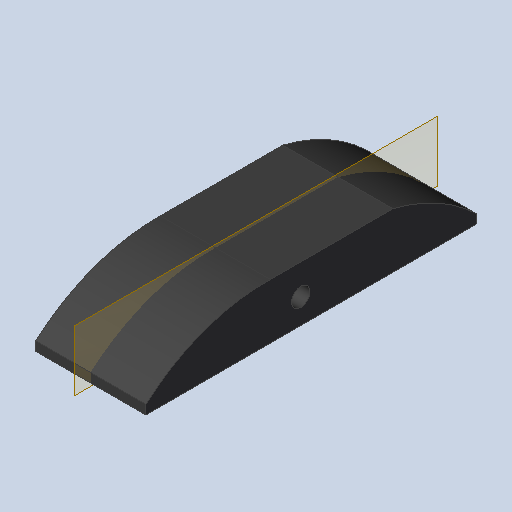
# Autodesk Inventor part: WingBox
Saved by Autodesk Inventor 2025.2 (Build 292293000, 293)
## iProperties
Created: 2025-02-16
Part Number: WingBox
Material: Generic
Document SubType Name: Modeling
Designer: Cupri
Density: 1 g/cm^3
Appearance: Default
Author: Cupri
Autodesk Inventor part; units mm, degrees
ref_plane "YZ Plane" through (0, 0, 0) normal (1, 0, 0) x (0, 1, 0)
ref_plane "XZ Plane" through (0, 0, 0) normal (0, 1, 0) x (-1, 0, 0)
ref_plane "XY Plane" through (0, 0, 0) normal (0, 0, 1) x (1, 0, 0)
sketch "Sketch1" plane through (0, 0, 0) normal (1, 0, 0) x (0, 1, 0)
  line L0 (-38.1, -165.1) -> (-38.1, 165.1)
  line L1 (-38.1, 165.1) -> (20.949, 165.1)
  line L2 (38.1, 77.5498) -> (38.1, -100.5752)
  line L3 (12.4566, -165.1) -> (-38.1, -165.1)
  line L4 (-38.1, -165.1) -> (38.1, 165.1) construction
  line L5 (-38.1, 165.1) -> (38.1, -165.1) construction
  line L6 (-38.1, -165.1) -> (-38.1, -215.9)
  line L7 (-38.1, -215.9) -> (-25.4, -215.9)
  line L8 (-25.4, -215.9) -> (-25.4, -165.1)
  line L9 (-38.1, 165.1) -> (-38.1, 241.3)
  line L10 (-38.1, 241.3) -> (-25.4, 241.3)
  line L11 (-25.4, 241.3) -> (-25.4, 165.1)
  line L12 (-38.1, -139.7) -> (38.1, -139.7) construction
  line L13 (-38.1, 12.7) -> (38.1, 12.7) construction
  line L14 (-38.1, 165.1) -> (38.1, 165.1) construction
  arc A0 (38.1, 68.9574) -> (-25.4, 241.3) centre (-215.8637, 73.2536) ccw
  arc A1 (-25.4, -215.9) -> (38.1, -100.5752) centre (-208.549, -39.9101) ccw
  point P0 (0, 0)
  dimension "d0" = 330.2
  dimension "d1" = 76.2
  dimension "d2" = 50.8
  dimension "d3" = 12.7
  dimension "d5" = 76.2
  dimension "d6" = 12.7
  dimension "d9" = 152.4
  dimension "d10" = 76.2
  dimension "d11" = 152.4
  dimension "d37" = 254
  dimension "d38" = 254
  constraints: 30 end point, 9 point on line, 8 perpendicular, 7 point on circle, 2 centre point, 2 midpoint, 2 parallel, 2 vertical
  measures "d0" distance of L0.start L0.end
  measures "d1" distance of L0.end L4.end
  measures "d2" distance of L0.start L6.end
  measures "d3" distance of L6.end L7.end
  measures "d5" distance of L0.end L9.end
  measures "d6" distance of L9.end L10.end
  measures "d9" distance between parallel lines of L13 L12
  measures "d10" distance from line of L12 L6.end
  measures "d11" distance between parallel lines of L14 L13
  measures "d37" radius of A0
  measures "d38" radius of A1
extrude "Extrusion1" add sketch "Sketch1" along normal mid plane 152.4
sketch "Sketch3" plane through (-76.2, -38.1, -215.9) normal (0, -1, 0) x (1, 0, 0)
  circle A0 centre (6.35, 76.2) radius 2.9972
  line L0 (0, 0) -> (0, 457.2) projected
  line L1 (0, 0) -> (152.4, 0) projected
  circle A1 centre (146.05, 76.2) radius 2.9972
  circle A2 centre (6.35, 228.6) radius 2.9972
  circle A3 centre (146.05, 228.6) radius 2.9972
  circle A4 centre (6.35, 381) radius 2.9972
  circle A5 centre (146.05, 381) radius 2.9972
  point P0 (76.2, 215.9)
  dimension "d14" = 5.9944
  dimension "d15" = 6.35
  dimension "d16" = 76.2
  dimension "d19" = 139.7
  dimension "d22" = 152.4
  constraints: 6 centre point, 1 horizontal, 1 vertical, 10 other
  measures "d14" diameter of A0
  measures "d15" distance from line of L0 A0.centre
  measures "d16" distance from line of L1 A0.centre
  measures "d19" distance of A0.centre A1.centre
  measures "d22" distance of A0.centre A2.centre
extrude "Extrusion2" cut sketch "Sketch3" against normal blind 12.7
ref_plane "Work Plane1" through (0, 0, 0) normal (1, 0, 0) x (0, 0, -1)
sketch "Sketch5" plane through (-76.2, 0, 0) normal (-1, 0, 0) x (0, 0, 1)
  ellipse E0 centre (75.0549, 61.9343) end of major axis (61.8185, 59.4799) minor radius 13.3797 projected
  point P0 (0, 0)
  constraints: 1 other
extrude "Extrusion4" cut sketch "Sketch5" against normal through all
sketch "Sketch6" plane through (-76.2, 0, 0) normal (-1, 0, 0) x (0, 0, 1)
  circle A0 centre (26.9178, -3.8046) radius 12.7
  point P0 (0, 0)
  dimension "d41" = 25.4
  constraints: 1 centre point
  measures "d41" diameter of A0
extrude "Extrusion5" cut sketch "Sketch6" against normal through all
body "Solid1"
